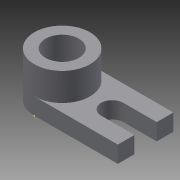
# Autodesk Inventor part: Locator
Saved by Autodesk Inventor 2015 (Build 190159000, 159)
## iProperties
Created: 2015-09-09
Part Number: Locator
Material: Generic
Document SubType Name: Modeling
Designer: Brandon
Density: 1 g/cm^3
Appearance: Default
Author: Brandon
Autodesk Inventor part; units mm, degrees
ref_plane "YZ Plane" through (0, 0, 0) normal (1, 0, 0) x (0, 1, 0)
ref_plane "XZ Plane" through (0, 0, 0) normal (0, 1, 0) x (-1, 0, 0)
ref_plane "XY Plane" through (0, 0, 0) normal (0, 0, 1) x (1, 0, 0)
sketch "Sketch1" plane through (0, 0, 0) normal (0, 0, 1) x (1, 0, 0)
  point P0 (0, 0)
sketch "Sketch2" plane through (0, 0, 0) normal (0, 0, 1) x (1, 0, 0)
  line L0 (0, 0) -> (75, 0)
  line L1 (75, 0) -> (75, 50)
  line L2 (75, 50) -> (0, 50)
  line L3 (0, 50) -> (0, 0)
  dimension "d0" = 75
  dimension "d1" = 50
  constraints: 8 end point, 2 parallel, 1 horizontal, 1 perpendicular
  measures "d0" distance of L2.end L1.end
  measures "d1" distance of L0.end L1.end
extrude "Extrusion1" add sketch "Sketch2" along normal blind 15
sketch "Sketch3" plane through (0, 0, 0) normal (0, 0, -1) x (-1, 0, 0)
  line L0 (0, 50) -> (0, 0) projected
  circle A0 centre (0, 25) radius 25
  constraints: 1 midpoint, 1 vertical alignment, 2 other
extrude "Extrusion2" add sketch "Sketch3" against normal blind 40
sketch "Sketch4" plane through (0, 25, 40) normal (0, 0, 1) x (1, 0, 0)
  circle A0 centre (0, 0) radius 25 projected
  circle A1 centre (0, 0) radius 15
  point P0 (0, -25)
  dimension "d6" = 30
  constraints: 1 centre point, 1 coincident, 1 vertical alignment
  measures "d6" diameter of A1
extrude "Extrusion3" cut sketch "Sketch4" against normal through all contours A1
hole "Hole1" at (45, 25, 15) direction (0, 0, -1) diameter 20 end through all
sketch "Sketch5" plane through (75, 0, 0) normal (1, 0, 0) x (0, 0, -1)
  line L0 (0, 15) -> (-15, 15)
  line L1 (-15, 15) -> (0, 15)
  line L2 (0, 15) -> (0, 35)
  line L3 (0, 35) -> (-15, 35)
  line L4 (-15, 35) -> (-15, 15)
  dimension "d19" = 20
  dimension "d20" = 15
  constraints: 10 end point, 2 parallel, 1 horizontal, 1 perpendicular
  measures "d19" distance of L2.end L1.end
  measures "d20" distance of L2.end L3.end
extrude "Extrusion4" cut sketch "Sketch5" against normal up to next
body "Solid1"
